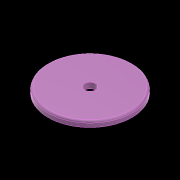
# Autodesk Inventor part: New Hub for old blade Lid
Saved by Autodesk Inventor 2022 (Build 260153000, 153)
## iProperties
Created: 2022-07-28
Part Number: New Hub for old blade Lid
Material: Custom TPU
Document SubType Name: Modeling
Designer: tandu
Density: 1.21 g/cm^3
Appearance: Smooth - Purple
Author: tandu
Autodesk Inventor part; units mm, degrees
ref_plane "YZ Plane" through (0, 0, 0) normal (1, 0, 0) x (0, 1, 0)
ref_plane "XZ Plane" through (0, 0, 0) normal (0, 1, 0) x (-1, 0, 0)
ref_plane "XY Plane" through (0, 0, 0) normal (0, 0, 1) x (1, 0, 0)
sketch "Sketch1" plane through (0, 0, 0) normal (0, 1, 0) x (-1, 0, 0)
  circle A0 centre (0, 0) radius 2.5
  circle A1 centre (0, 0) radius 18.9236
  dimension "d0" = 5
  dimension "d1" = 37.8473
  constraints: 2 centre point, 2 coincident
  measures "d0" diameter of A0
  measures "d1" diameter of A1
extrude "Extrusion1" add sketch "Sketch1" along normal blind 2.54
fillet "Fillet1" radius 0.7937 1 edges at (18.9236, 2.54, 0)
body "Solid1"
